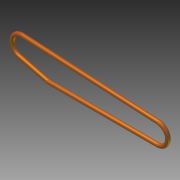
# Autodesk Inventor part: apendage polycord
Saved by Autodesk Inventor 2012 (Build 160160000, 160)
## iProperties
Created: 2013-07-07
Part Number: apendage polycord
Material: Default
Document SubType Name: Modeling
Designer: Bryce
Density: 1 g/cm^3
Author: Bryce
Autodesk Inventor part; units mm, degrees
ref_plane "YZ Plane" through (0, 0, 0) normal (1, 0, 0) x (0, 1, 0)
ref_plane "XZ Plane" through (0, 0, 0) normal (0, 1, 0) x (-1, 0, 0)
ref_plane "XY Plane" through (0, 0, 0) normal (0, 0, 1) x (1, 0, 0)
sketch "Sketch1" plane through (0, 0, 0) normal (0, 0, 1) x (1, 0, 0)
  arc A0 (0, -15.875) -> (0.8198, 15.8538) centre (0, 0) ccw
  line L0 (0, -15.875) -> (-171.45, -15.875)
  arc A1 (-175.3175, -15.3967) -> (-171.45, -15.875) centre (-171.45, 0) ccw
  line L1 (-175.3175, -15.3967) -> (-219.7585, -4.2334)
  arc A2 (-215.0712, 27.0171) -> (-219.7585, -4.2334) centre (-215.891, 11.1633) ccw
  line L2 (-215.0712, 27.0171) -> (0.8198, 15.8538)
  dimension "d0" = 171.45
  dimension "d1" = 15.875
  dimension "d2" = 45.8216
  dimension "d3" = 216.1794
  dimension "d4" = 15.875
  dimension "d5" = 15.875
  constraints: 6 end point, 6 point on circle, 6 tangent, 3 centre point, 1 coincident, 1 horizontal
  measures "d0" distance of L0.start L0.end
  measures "d1" radius of A0
  measures "d2" distance of L1.start L1.end
  measures "d3" distance of L2.start L2.end
  measures "d4" radius of A2
  measures "d5" radius of A1
sketch "Sketch2" plane through (0, 0, 0) normal (1, 0, 0) x (0, 1, 0)
  circle A0 centre (-15.875, 0) radius 3.175
  point P0 (0, 0)
  dimension "d6" = 15.875
  dimension "d7" = 6.35
  constraints: 1 centre point, 1 horizontal alignment
  measures "d6" distance of A0.centre point (0, 0)
  measures "d7" diameter of A0
sweep "Sweep1" add profiles "Sketch2" path "Sketch1"
equation "\"d4\" = d1"
equation "\"d5\" = d1"
body "Solid1"
